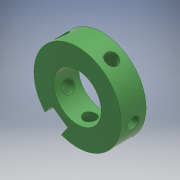
# Autodesk Inventor part: sprzeglo_04
Saved by Autodesk Inventor 2017 (Build 210142000, 142)
## iProperties
Created: 2021-05-22
Part Number: sprzeglo_04
Material: Generic
Document SubType Name: Modeling
Designer: majch
Density: 1 g/cm^3
Appearance: Smooth - Dark Forest Green
Author: majch
Autodesk Inventor part; units mm, degrees
ref_plane "YZ Plane" through (0, 0, 0) normal (1, 0, 0) x (0, 1, 0)
ref_plane "XZ Plane" through (0, 0, 0) normal (0, 1, 0) x (-1, 0, 0)
sketch "Sketch1" plane through (0, 0, 0) normal (0, 1, 0) x (-1, 0, 0)
  circle A0 centre (0, 0) radius 17.5
  dimension "d0" = 35
  constraints: 1 centre point, 1 coincident
  measures "d0" diameter of A0
extrude "Extrusion1" add sketch "Sketch1" along normal blind 10
sketch "Sketch2" plane through (0, 10, 0) normal (0, 1, 0) x (1, 0, 0)
  circle A0 centre (0, 0) radius 9.5
  dimension "d3" = 19
  constraints: 1 centre point, 1 coincident
  measures "d3" diameter of A0
extrude "Extrusion2" cut sketch "Sketch2" against normal through all
ref_plane "Work Plane13" through (0, 0, 0) normal (0, 0, 1) x (0, 1, 0)
sketch "Sketch11" plane through (0, 0, 0) normal (0, 0, 1) x (0, 1, 0)
  circle A0 centre (5, 0) radius 2.5
  point P0 (0, 0)
  dimension "d52" = 5
  constraints: 1 centre point
  measures "d52" diameter of A0
hole "Hole5" at (0, 5, 0) direction (0, 0, -1) diameter 5 end through all
ref_plane "Work Plane14" through (0, 0, 0) normal (0.9396926, 0, 0.3420201) x (0, 1, 0)
sketch "Sketch12" plane through (0, 0, 0) normal (0.9396926, 0, 0.3420201) x (0, 1, 0)
  circle A0 centre (5, 0) radius 2.5
  point P0 (0, 0)
  dimension "d61" = 5
  constraints: 1 centre point
  measures "d61" diameter of A0
hole "Hole6" at (0, 5, 0) direction (-0.9396926, 0, -0.3420201) diameter 5 end through all
ref_plane "Work Plane15" through (0, 0, 0) normal (0.6427876, 0, -0.7660444) x (0, 1, 0)
sketch "Sketch13" plane through (0, 0, 0) normal (0.6427876, 0, -0.7660444) x (0, 1, 0)
  circle A0 centre (5, 0) radius 2.5
  point P0 (0, 0)
  dimension "d70" = 5
  constraints: 1 centre point
  measures "d70" diameter of A0
hole "Hole7" at (0, 5, 0) direction (-0.6427876, 0, 0.7660444) diameter 5 end through all
ref_plane "Work Plane16" through (0, 0, 0) normal (-0.5, 0, -0.8660254) x (0, 1, 0)
sketch "Sketch14" plane through (0, 0, 0) normal (-0.5, 0, -0.8660254) x (0, 1, 0)
  circle A0 centre (5, 0) radius 2.5
  point P0 (0, 0)
  dimension "d79" = 5
  constraints: 1 centre point
  measures "d79" diameter of A0
hole "Hole8" at (0, 5, 0) direction (0.5, 0, 0.8660254) diameter 5 end through all
ref_plane "Work Plane17" through (0, 0, 0) normal (-0.9848078, 0, 0.1736482) x (0, 1, 0)
sketch "Sketch15" plane through (0, 0, 0) normal (-0.9848078, 0, 0.1736482) x (0, 1, 0)
  circle A0 centre (5, 0) radius 2.5
  point P0 (0, 0)
  dimension "d88" = 5
  constraints: 1 centre point
  measures "d88" diameter of A0
hole "Hole9" at (0, 5, 0) direction (0.9848078, 0, -0.1736482) diameter 5 end through all
ref_plane "Work Plane21" through (-10.0376, 0, -14.3352) normal (0.5735764, 0, 0.819152) x (0, 1, 0)
ref_plane "Work Plane20" through (0, 0, 0) normal (0.5735764, 0, 0.819152) x (0, 1, 0)
sketch "Sketch16" plane through (-10.0376, 0, -14.3352) normal (0.5735764, 0, 0.819152) x (0, 1, 0)
  line L0 (10, 4) -> (0, 4)
  line L1 (0, 4) -> (0, -4)
  line L2 (0, -4) -> (10, -4)
  line L3 (10, -4) -> (10, 4)
  line L4 (0, 17.5) -> (0, -17.5)
  line L5 (18.3389, 0) -> (-7, 0) construction
  point P0 (0, 0)
  dimension "d100" = 8
  dimension "d107" = 4
  dimension "d108" = 10
  constraints: 12 end point, 2 horizontal, 2 parallel, 1 perpendicular
  measures "d100" distance of L0.end L1.end
  measures "d107" distance between parallel lines of L5 L2
  measures "d108" distance of L0.start L0.end
extrude "Extrusion4" cut sketch "Sketch16" along normal blind 5
equation "\"d107\" = 0.5 * d100"
body "Solid1"
